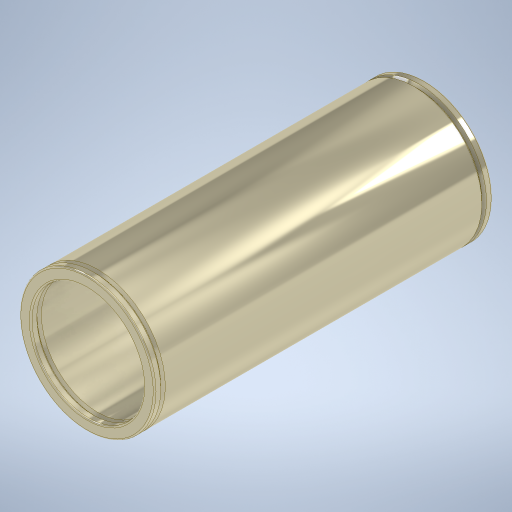
# Autodesk Inventor part: IFL
Saved by Autodesk Inventor 2023 (Build 270158000, 158)
## iProperties
RuleStatus: InUse
Created: 2022-07-07
Part Number: IFL
Material: Generic
Document SubType Name: Modeling
Designer: Admin
Density: 1 g/cm^3
Appearance: Nickel
Author: Admin
Autodesk Inventor part; units mm, degrees
ref_plane "YZ Plane" through (0, 0, 0) normal (1, 0, 0) x (0, 1, 0)
ref_plane "XZ Plane" through (0, 0, 0) normal (0, 1, 0) x (-1, 0, 0)
ref_plane "XY Plane" through (0, 0, 0) normal (0, 0, 1) x (1, 0, 0)
sketch "Profile Sketch" plane through (0, 0, 0) normal (1, 0, 0) x (0, 1, 0)
  line L0 (0, 381) -> (0, -381)
  line L1 (127, 381) -> (152.4, 381)
  line L2 (152.4, 381) -> (152.4, 361.95)
  line L3 (127, 381) -> (127, 361.95)
  line L4 (146.05, 361.95) -> (152.4, 361.95)
  line L5 (152.4, 361.95) -> (152.4, -361.95)
  line L6 (146.05, -361.95) -> (146.05, 361.95)
  line L7 (127, 361.95) -> (133.35, 361.95)
  line L8 (133.35, 361.95) -> (133.35, -361.95)
  line L9 (127, -361.95) -> (127, 361.95)
  line L10 (127, 361.95) -> (133.35, 361.95)
  line L11 (133.35, 361.95) -> (133.35, 360.045)
  line L12 (152.4, 361.95) -> (146.05, 361.95)
  line L13 (146.05, 361.95) -> (146.05, 360.045)
  line L14 (146.05, 360.045) -> (133.35, 360.045)
  line L15 (127, -361.95) -> (133.35, -361.95)
  line L16 (146.05, -361.95) -> (152.4, -361.95)
  line L17 (127, -381) -> (152.4, -381)
  line L18 (152.4, -381) -> (152.4, -361.95)
  line L19 (127, -381) -> (127, -361.95)
  line L20 (127, -361.95) -> (133.35, -361.95)
  line L21 (133.35, -361.95) -> (133.35, -360.045)
  line L22 (152.4, -361.95) -> (146.05, -361.95)
  line L23 (133.35, -360.045) -> (146.05, -360.045)
  line L24 (146.05, -360.045) -> (146.05, -361.95)
  point P0 (0, 0)
  point P1 (0, 0)
  point P2 (152.4, 0)
  point P3 (127, 0)
  point P4 (133.35, -360.045)
  dimension "tubeLength" = 762
  dimension "outerTubeOd" = 304.8
  dimension "innerTubeId" = 254
  dimension "d18" = 1.905
  dimension "endCapThickness" = 19.05
  dimension "d22" = 292.1
  dimension "d23" = 266.7
  constraints: 50 end point, 12 perpendicular, 8 horizontal, 4 collinear, 4 equal length, 3 horizontal alignment, 3 midpoint, 2 parallel, 1 coincident, 1 point on line, 1 vertical
  measures "tubeLength" distance of L0.start L0.end
  measures "outerTubeOd" diameter of L5 L0
  measures "innerTubeId" diameter of L9 L0
  measures "d18" distance of L7.end L11.end
  measures "endCapThickness" distance of L1.start L3.end
  measures "d22" diameter of L6 L0
  measures "d23" diameter of L8 L0
revolve "Inner Tube Revolution" add sketch "Profile Sketch" angle 360 about axis through (0, 0, 381) along (0, 0, -1) contours L5 L16 L6 L4
revolve "Outer Tube Revolution" add sketch "Profile Sketch" angle 360 about axis through (0, 0, 381) along (0, 0, -1) separate body contours L7 L8 L15 L9
revolve "Front End Cap Revolution" add sketch "Profile Sketch" angle 360 about axis through (0, 0, 381) along (0, 0, -1) separate body contours L1 L2 L4 L6 L14 L8 L7 L3
revolve "Back End Cap Revolution" add sketch "Profile Sketch" angle 360 about axis through (0, 0, 381) along (0, 0, -1) separate body contours L15 L8 L23 L6 L16 L18 L17 L19
fillet "Fillet1" radius 3.175 4 edges at (0, -127, 381) (0, -152.4, 381) (0, -152.4, -381) (0, -127, -381)
chamfer "Chamfer1" distance 5.08 angle 45 4 edges at (0, -152.4, 361.95) (0, -152.4, -361.95) (0, -127, -361.95) (0, -127, 361.95)
equation "\"d22\" = outerTubeOd - 2 * tubeThickness"
equation "\"d23\" = innerTubeId + 2 * tubeThickness"
equation "\"tubeThickness\" = 6.35"
